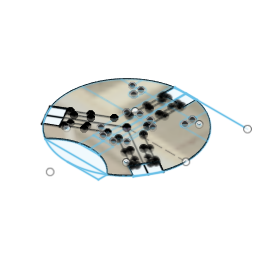
BaseChapaBaixo+Draw (Autodesk Fusion 360 archive; units mm, degrees)
design "BaseChapaBaixo"
Autodesk Fusion 360 part; units mm, degrees
sketch "Sketch1" plane through (0, 0, 0) normal (0, 1, 0) x (1, 0, 0)
  circle A0 centre (0, 0) radius 240
  line L0 (0, -240) -> (125, -240)
  line L1 (125, -240) -> (125, -204.878)
  line L2 (0, 240) -> (0, -147)
  line L3 (125, -204.878) -> (-125, -204.878)
  arc A1 (125, -204.878) -> (-125, -204.878) centre (0, -310.9212) ccw
  circle A2 centre (-53.8749, 53.8749) radius 5
  line L4 (-53.8749, 53.8749) -> (51.1251, 53.8749)
  line L5 (51.1251, 53.8749) -> (51.1251, -51.1251)
  line L6 (51.1251, -51.1251) -> (-53.8749, -51.1251)
  line L7 (-53.8749, -51.1251) -> (-53.8749, 53.8749)
  circle A3 centre (51.1251, 53.8749) radius 5
  circle A4 centre (51.1251, -51.1251) radius 5
  circle A5 centre (-53.8749, -51.1251) radius 5
  line L8 (0, 240) -> (250, 240)
  line L9 (-53.8749, 53.8749) -> (-53.8749, 233.8749)
  line L10 (-53.8749, 53.8749) -> (-233.8749, 53.8749)
  line L11 (105.2845, 215.6738) -> (105.2845, 175.6738)
  line L12 (105.2845, 175.6738) -> (105.2845, 115.6738)
  line L13 (105.2845, 115.6738) -> (210.2845, 115.6738)
  line L14 (105.2845, 115.6738) -> (105.2845, 130.6738)
  line L15 (105.2845, 175.6738) -> (105.2845, 160.6738)
  line L16 (120.2845, 130.6738) -> (120.2845, 160.6738)
  arc A6 (120.2845, 160.6738) -> (90.2845, 160.6738) centre (105.2845, 160.6738) ccw
  line L17 (90.2845, 160.6738) -> (90.2845, 130.6738)
  arc A7 (90.2845, 130.6738) -> (120.2845, 130.6738) centre (105.2845, 130.6738) ccw
  line L18 (105.2845, 130.6738) -> (105.2845, 160.6738) construction
  line L19 (0, -147) -> (40, -147)
  line L20 (40, -147) -> (40, -151.9553)
  line L21 (0, -147) -> (0, -95)
  line L22 (0, -95) -> (-40, -95)
  line L23 (40, -151.9553) -> (-40, -151.9553)
  line L24 (-40, -151.9553) -> (-40, -95)
  line L25 (-40, -95) -> (40, -95)
  line L26 (40, -95) -> (40, -151.9553)
  line L27 (-135.688, 197.9615) -> (-135.688, 157.9615)
  line L28 (-135.688, 157.9615) -> (-180.688, 157.9615)
  circle A8 centre (-135.688, 157.9615) radius 5
  line L29 (-135.688, 157.9615) -> (-102.688, 157.9615)
  line L30 (105.2845, 160.6738) -> (-102.688, 160.6738)
  line L31 (-102.688, 160.6738) -> (-102.688, 130.6738)
  line L32 (-117.688, 160.6738) -> (-117.688, 130.6738)
  arc A9 (-117.688, 130.6738) -> (-87.688, 130.6738) centre (-102.688, 130.6738) ccw
  line L33 (-87.688, 130.6738) -> (-87.688, 160.6738)
  arc A10 (-87.688, 160.6738) -> (-117.688, 160.6738) centre (-102.688, 160.6738) ccw
  line L34 (-102.688, 160.6738) -> (-102.688, 130.6738) construction
  line L35 (-102.688, 157.9615) -> (-102.688, 160.6738)
  line L36 (0, 0) -> (207.8461, -120)
  line L37 (0, 0) -> (240, 0) construction
  line L38 (0, 0) -> (-207.8461, -120)
  line L39 (0, 0) -> (0, 240)
  line L40 (0, 240) -> (45, 240)
  line L41 (45, 240) -> (-45, 240)
  line L42 (-45, 240) -> (-45, 187)
  line L43 (-45, 187) -> (45, 187)
  line L44 (45, 187) -> (45, 240)
  line L45 (207.8461, -120) -> (185.3461, -158.9711)
  line L46 (207.8461, -120) -> (230.3461, -81.0289)
  line L47 (230.3461, -81.0289) -> (184.4468, -54.5289)
  line L48 (184.4468, -54.5289) -> (139.4468, -132.4711)
  line L49 (139.4468, -132.4711) -> (185.3461, -158.9711)
  line L50 (-207.8461, -120) -> (-185.3461, -158.9711)
  line L51 (-185.3461, -158.9711) -> (-139.4468, -132.4711)
  line L52 (-139.4468, -132.4711) -> (-184.4468, -54.5289)
  line L53 (-184.4468, -54.5289) -> (-230.3461, -81.0289)
  line L54 (-207.8461, -120) -> (-230.3461, -81.0289)
  line L55 (-40, -95) -> (-40, -75)
  line L56 (-40, -75) -> (40, -75)
  line L57 (40, -75) -> (40, 74)
  line L58 (40, 74) -> (-40, 74)
  line L59 (0, -75) -> (21, -75)
  line L60 (21, -75) -> (-21, -75)
  line L61 (-21, -75) -> (-21, 74)
  line L62 (21, -75) -> (21, 74)
  circle A11 centre (-21, 74) radius 2
  circle A12 centre (21, 74) radius 2
  circle A13 centre (-21, -75) radius 2
  circle A14 centre (21, -75) radius 2
  line L63 (-139.4468, -132.4711) -> (-143.4468, -125.5429)
  line L64 (-184.4468, -54.5289) -> (-180.4468, -61.4571)
  line L65 (-143.4468, -125.5429) -> (-134.7865, -120.5429)
  line L66 (-134.7865, -120.5429) -> (-82.825, -90.5429)
  line L67 (-82.825, -90.5429) -> (-22.2032, -55.5429)
  line L68 (-139.4468, -132.4711) -> (-151.9468, -110.8205)
  line L69 (-151.9468, -110.8205) -> (-130.2961, -98.3205)
  line L70 (-130.2961, -98.3205) -> (-86.9948, -73.3205)
  line L71 (-184.4468, -54.5289) -> (-171.9468, -76.1795)
  line L72 (-171.9468, -76.1795) -> (-150.2961, -63.6795)
  line L73 (-150.2961, -63.6795) -> (-106.9948, -38.6795)
  line L74 (-180.4468, -61.4571) -> (-171.7865, -56.4571)
  line L75 (-171.7865, -56.4571) -> (-119.825, -26.4571)
  line L76 (-119.825, -26.4571) -> (-59.2032, 8.5429)
  circle A15 centre (-22.2032, -55.5429) radius 2.5
  circle A16 centre (-82.825, -90.5429) radius 2.5
  circle A17 centre (-134.7865, -120.5429) radius 2.5
  circle A18 centre (-59.2032, 8.5429) radius 2.5
  circle A19 centre (-119.825, -26.4571) radius 2.5
  circle A20 centre (-171.7865, -56.4571) radius 2.5
  circle A21 centre (-106.9948, -38.6795) radius 2.5
  circle A22 centre (-150.2961, -63.6795) radius 2.5
  circle A23 centre (-86.9948, -73.3205) radius 2.5
  circle A24 centre (-130.2961, -98.3205) radius 2.5
  circle A25 centre (59.2032, 8.5429) radius 2.5
  circle A26 centre (119.825, -26.4571) radius 2.5
  circle A27 centre (171.7865, -56.4571) radius 2.5
  circle A28 centre (150.2961, -63.6795) radius 2.5
  line L77 (150.2961, -63.6795) -> (106.9948, -38.6795)
  circle A29 centre (106.9948, -38.6795) radius 2.5
  circle A30 centre (130.2961, -98.3205) radius 2.5
  circle A31 centre (86.9948, -73.3205) radius 2.5
  circle A32 centre (82.825, -90.5429) radius 2.5
  circle A33 centre (134.7865, -120.5429) radius 2.5
  circle A34 centre (22.2032, -55.5429) radius 2.5
  line L78 (82.825, -90.5429) -> (22.2032, -55.5429)
  line L79 (134.7865, -120.5429) -> (82.825, -90.5429)
  line L80 (143.4468, -125.5429) -> (134.7865, -120.5429)
  line L81 (151.9468, -110.8205) -> (130.2961, -98.3205)
  line L82 (130.2961, -98.3205) -> (86.9948, -73.3205)
  line L83 (171.9468, -76.1795) -> (150.2961, -63.6795)
  line L84 (180.4468, -61.4571) -> (171.7865, -56.4571)
  line L85 (171.7865, -56.4571) -> (119.825, -26.4571)
  line L86 (119.825, -26.4571) -> (59.2032, 8.5429)
  circle A35 centre (-37, 47) radius 2.5
  circle A36 centre (-37, 117) radius 2.5
  circle A37 centre (-37, 177) radius 2.5
  circle A38 centre (-20, 162) radius 2.5
  line L87 (-20, 162) -> (-20, 112)
  circle A39 centre (-20, 112) radius 2.5
  circle A40 centre (20, 162) radius 2.5
  circle A41 centre (20, 112) radius 2.5
  circle A42 centre (37, 117) radius 2.5
  circle A43 centre (37, 177) radius 2.5
  circle A44 centre (37, 47) radius 2.5
  line L88 (37, 117) -> (37, 47)
  line L89 (37, 177) -> (37, 117)
  line L90 (37, 187) -> (37, 177)
  line L91 (20, 187) -> (20, 162)
  line L92 (20, 162) -> (20, 112)
  line L93 (-20, 187) -> (-20, 162)
  line L94 (-37, 187) -> (-37, 177)
  line L95 (-37, 177) -> (-37, 117)
  line L96 (-37, 117) -> (-37, 47)
  circle A45 centre (135.688, 157.9615) radius 5
  circle A46 centre (120.8737, -122.997) radius 5
  circle A47 centre (-120.8737, -122.997) radius 5
  point P0 (-106.9948, -38.6795)
  point P1 (-150.2961, -63.6795)
  point P2 (-59.2032, 8.5429)
  point P3 (-119.825, -26.4571)
  point P4 (-171.7865, -56.4571)
  dimension "d2" = 125
  dimension "d3" = 387
  dimension "d7" = 10
  dimension "d8" = 105
  dimension "d9" = 105
  dimension "d10" = 10
  dimension "d11" = 10
  dimension "d12" = 10
  dimension "d13" = 250
  dimension "d14" = 180
  dimension "d15" = 180
  dimension "d16" = 40
  dimension "d17" = 60
  dimension "d18" = 105
  dimension "d19" = 15
  dimension "d20" = 15
  dimension "d21" = 30
  dimension "d22" = 40
  dimension "d23" = 52
  dimension "d24" = 40
  dimension "d25" = 40
  dimension "d26" = 45
  dimension "d27" = 10
  dimension "d28" = 33
  dimension "d29" = 30
  dimension "d30" = 30
  dimension "d40" = 30
  dimension "d41" = 60
  dimension "d42" = 240
  dimension "d46" = 45
  dimension "d47" = 90
  dimension "d48" = 53
  dimension "d49" = 45
  dimension "d50" = 45
  dimension "d53" = 45
  dimension "d54" = 53
  dimension "d55" = 90
  dimension "d56" = 53
  dimension "d57" = 20
  dimension "d58" = 80
  dimension "d59" = 149
  dimension "d60" = 80
  dimension "d61" = 21
  dimension "d62" = 42
  dimension "d63" = 4
  dimension "d64" = 4
  dimension "d65" = 4
  dimension "d66" = 4
  dimension "d67" = 8
  dimension "d68" = 8
  dimension "d69" = 10
  dimension "d70" = 60
  dimension "d71" = 70
  dimension "d72" = 25
  dimension "d73" = 25
  dimension "d74" = 50
  dimension "d75" = 25
  dimension "d76" = 5
  dimension "d77" = 5
  dimension "d78" = 5
  dimension "d79" = 5
  dimension "d80" = 5
  dimension "d81" = 5
  dimension "d82" = 5
  dimension "d83" = 5
  dimension "d84" = 5
  dimension "d85" = 5
  dimension "d87" = 360
  dimension "d33" = 10
  constraint coincident A0.centre L36.start
  constraint coincident A0 L0.start
  constraint horizontal L0
  constraint coincident A0 L1.end
  constraint perpendicular L0 L1
  constraint coincident A0 L2.start
  constraint vertical L2
  constraint coincident A0 L3.end
  constraint perpendicular L1 L3
  constraint coincident L2.end A1
  constraint horizontal L4
  constraint vertical L5
  constraint horizontal L6
  constraint vertical L7
  constraint coincident A2.centre L4.start
  constraint coincident L4.end L5.start
  constraint coincident L5.end L6.start
  constraint coincident L6.end L7.start
  constraint perpendicular L2 L8
  constraint coincident A0 L9.end
  constraint parallel L7 L9
  constraint coincident A0 L10.end
  constraint perpendicular L9 L10
  constraint coincident A0 L11.start
  constraint vertical L11
  constraint parallel L11 L12
  constraint perpendicular L12 L13
  constraint coincident A0 L13.end
  constraint perpendicular L13 L14
  constraint parallel L12 L15
  constraint tangent L16 A6
  constraint tangent A6 L17
  constraint parallel L16 L17
  constraint tangent L17 A7
  constraint tangent L16 A7
  constraint coincident L15.end A6.centre
  constraint parallel L15 L18
  constraint coincident L14.end A7.centre
  constraint perpendicular L2 L19
  constraint coincident A1 L20.end
  constraint perpendicular L19 L20
  constraint perpendicular L19 L21
  constraint perpendicular L2 L22
  constraint horizontal L23
  constraint vertical L24
  constraint horizontal L25
  constraint vertical L26
  constraint coincident A0 L27.start
  constraint parallel L2 L27
  constraint coincident A0 L28.end
  constraint perpendicular L27 L28
  constraint coincident L27.end L28.start
  constraint perpendicular L27 L29
  constraint perpendicular L15 L30
  constraint perpendicular L30 L31
  constraint tangent L32 A9
  constraint tangent A9 L33
  constraint parallel L32 L33
  constraint tangent L33 A10
  constraint tangent L32 A10
  constraint coincident L31.end A9.centre
  constraint perpendicular L29 L34
  constraint coincident L30.end L31.start
  constraint perpendicular L30 L35
  constraint horizontal L37
  constraint perpendicular L2 L40
  constraint horizontal L41
  constraint vertical L42
  constraint horizontal L43
  constraint vertical L44
  constraint perpendicular L36 L45
  constraint perpendicular L36 L46
  constraint perpendicular L46 L47
  constraint perpendicular L47 L48
  constraint perpendicular L38 L50
  constraint perpendicular L50 L51
  constraint perpendicular L51 L52
  constraint perpendicular L52 L53
  constraint perpendicular L25 L55
  constraint perpendicular L24 L56
  constraint perpendicular L6 L57
  constraint perpendicular L57 L58
  constraint midpoint L56 L59.start
  constraint perpendicular L2 L59
  constraint parallel L56 L60
  constraint coincident L58 L61.end
  constraint perpendicular L58 L61
  constraint coincident L58 L62.end
  constraint perpendicular L58 L62
  constraint coincident L61.end A11.centre
  constraint coincident L62.end A12.centre
  constraint coincident L60.end L61.start
  constraint coincident L59.end L60.start
  constraint perpendicular L51 L63
  constraint perpendicular L53 L64
  constraint perpendicular L63 L65
  constraint parallel L65 L66
  constraint parallel L66 L67
  constraint perpendicular L65 L68
  constraint perpendicular L68 L69
  constraint parallel L69 L70
  constraint symmetric L38 L69.end P1
  constraint symmetric L38 L70.end P0
  constraint perpendicular L53 L71
  constraint coincident P1 L72.end
  constraint coincident P0 L73.end
  constraint symmetric L38 L65.end P4
  constraint symmetric L38 L66.end P3
  constraint symmetric L38 L67.end P2
  constraint coincident P4 L74.end
  constraint coincident P3 L75.end
  constraint coincident P2 L76.end
  constraint coincident L67.end A15.centre
  constraint coincident L66.end L67.start
  constraint coincident L65.end L66.start
  constraint coincident L70.end A23.centre
  constraint coincident L69.end L70.start
  constraint symmetric L2 A8 A45
  measures "d2" distance of L0.start L0.end
  measures "d3" distance of L2.start L2.end
  measures "d7" diameter of A2
  measures "d8" distance of A2.centre L4.end
  measures "d9" distance of A2.centre L6.end
  measures "d10" diameter of A3
  measures "d11" diameter of A4
  measures "d12" diameter of A5
  measures "d13" distance of L2.start L8.end
  measures "d14" distance of A2.centre L10.end
  measures "d15" distance of A2.centre L9.end
  measures "d16" distance of L11.start L11.end
  measures "d17" distance of L11.end L12.end
  measures "d18" distance of L12.end L13.end
  measures "d19" distance of L12.end L14.end
  measures "d20" distance of L11.end L15.end
  measures "d21" diameter of A6
  measures "d22" distance of L2.end L19.end
  measures "d23" distance of L2.end L21.end
  measures "d24" distance of L21.end L22.end
  measures "d25" distance of L27.start L27.end
  measures "d26" distance of L27.end L28.end
  measures "d27" diameter of A8
  measures "d28" distance of L27.end L29.end
  measures "d29" distance of L30.end L31.end
  measures "d30" diameter of A9
  measures "d40" angle of L36 L37
  measures "d41" angle of L36 L38
  measures "d42" distance of A0.centre L38.end
  measures "d46" distance of L2.start L40.end
  measures "d47" distance of L40.end L41.end
  measures "d48" distance of L40.end L43.end
  measures "d49" distance of L36.end L45.end
  measures "d50" distance of L36.end L46.end
  measures "d53" distance of L38.end L50.end
  measures "d54" distance of L50.end L51.end
  measures "d55" distance of L51.end L52.end
  measures "d56" distance of L52.end L53.end
  measures "d57" distance of L22.end L55.end
  measures "d58" distance of L55.end L56.end
  measures "d59" distance of L56.end L57.end
  measures "d60" distance of L57.end L58.end
  measures "d61" distance of L59.start L59.end
  measures "d62" distance of L59.end L60.end
  measures "d63" diameter of A11
  measures "d64" diameter of A12
  measures "d65" diameter of A13
  measures "d66" diameter of A14
  measures "d67" distance of L51.end L63.end
  measures "d68" distance of L52.end L64.end
  measures "d69" distance of L63.end L65.end
  measures "d70" distance of L65.end L66.end
  measures "d71" distance of L66.end L67.end
  measures "d72" distance of L51.end L68.end
  measures "d73" distance of L68.end L69.end
  measures "d74" distance of L69.end L70.end
  measures "d75" distance of L52.end L71.end
  measures "d76" diameter of A15
  measures "d77" diameter of A16
  measures "d78" diameter of A17
  measures "d79" diameter of A18
  measures "d80" diameter of A19
  measures "d81" diameter of A20
  measures "d82" diameter of A21
  measures "d83" diameter of A22
  measures "d84" diameter of A23
  measures "d85" diameter of A24
  measures "d33" diameter of A47
extrude "Extrude1" add sketch "Sketch1" along normal blind 3 contours A0 L4 L5 A3 L13 L17 A7 L30 L36 L47 L48 L57 L58 A42 L88 L89 | A0 L11 L13 L16 A6 A7 | A0 L11 A6 L30 L43 L44 A43 L89 L90 | L12 L14 L17 A7 L30 | L12 L14 L15 L16 A6 A7 | L12 L15 A6 L30 | A0 L2 A1 L20 L25 L26 L48 L49 L56 L57 L59 L60 A14 A32 A33 L78 L79 L80 | L5 L6 A4 L36 L48 L57 A32 A33 L78 L79 L80 | L4 L5 A3 L36 L57 | L5 L6 A4 L36 L57 | A0 L9 L30 L42 L43 A37 L94 L95 | L2 L30 L39 L43 A40 L91 | L2 L30 L39 L43 A38 L93 | L30 L43 A40 A43 L89 L90 L91 | L2 L30 L39 L58 A12 A40 A42 L88 L89 | A0 A1 L24 L51 L52 L55 L56 L61 A13 L63 L65 L66 L67 L68 A15 A16 A17 | A1 L19 L20 L26 | L4 L5 A3 | L4 L5 A3 | L5 L6 A4 | L5 L6 A4 | L6 L36 L57 L62 | L4 L36 L57 L62 | A0 L9 L27 A8 L29 L30 L32 A10 | L2 L30 L39 L58 A11 A36 A38 L95 L96 | L30 L43 A37 A38 L93 L94 L95 | L30 A40 L92 | L30 A40 L91 L92 | L2 A1 L21 L22 L24 L25 | L2 L19 L21 L25 L26 | L2 L6 L36 L62 | L2 L4 L36 L39 L62 | L6 L57 L62 A34 L78 | L4 L57 L58 L88 | A0 L27 L28 A8 | A2 L4 L9 L30 A36 L95 L96 | A0 A2 L9 L10 L28 A8 L29 L30 L32 A9 L33 | L2 L4 L39 L58 L62 A12 | L2 L4 L39 L58 L61 A11 | L30 A40 L91 L92 | L30 A40 L92 | L30 A38 L87 | L30 A38 L87 L93 | L30 A38 L87 L93 | L2 L22 L25 L55 L56 L60 A13 | L2 L4 L38 L39 L61 | L2 L6 L38 L61 | L2 L6 L56 L59 L60 L62 A14 A34 | L4 L58 L62 A12 L88 | L56 L57 L62 A14 A34 L78 | A2 L9 L10 | A2 L4 L9 | L29 L30 L31 L32 A9 L33 L35 | L29 L30 L31 L32 A10 L35 | L58 A12 | L58 L62 A12 | L58 L61 A11 | L58 A11 | L30 A38 L87 | A0 A2 L7 L10 L38 L52 L53 L64 L71 | L6 L7 A5 L38 L52 L61 L65 L66 L67 L68 A15 A16 A17 | L2 L6 L56 L60 L61 A13 A15 | L6 L7 A5 L38 L61 | A2 L4 L7 L38 L61 | L58 L62 A12 | A2 L4 L7 | A2 L7 L10 | L4 L58 L61 A11 L96 | L58 L61 A11 | L56 L61 A13 | L56 L60 A13 | L56 L60 L61 A13 | L56 L59 L60 L62 A14 | L56 L59 L60 A14 | L56 L62 A14 | L6 L7 A5 | L6 L7 A5 | L69 L70 A24 | L69 L70 A24 | L72 L73 A22 | L72 L73 A22 | A21 | A23 | A28 L77 L83 | A28 L77 L83 | A29 | A30 L81 L82 | A30 L81 L82 | A31 | A39 | A41
move_body "Move1" [rolled back]
equation "d2 = ( 250 / 2 ) * 1 mm"
equation "d3 = 355 mm + 32 mm"
equation "d61 = ( 42 / 2 ) * 1 mm"
